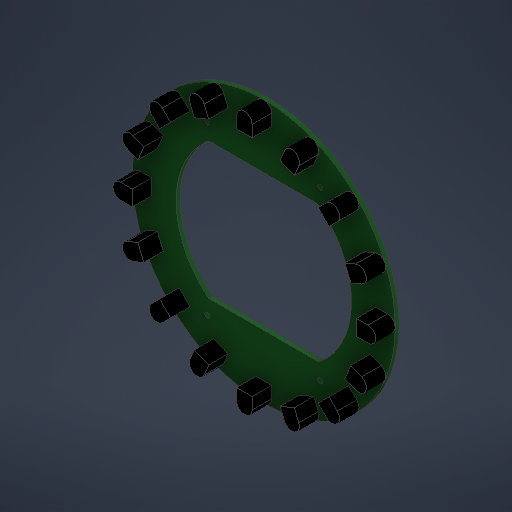
# Autodesk Inventor part: Main Board
Saved by Autodesk Inventor 2026.1 (Build 301233020, 233B)
## iProperties
Created: 2025-11-27
Part Number: Main Board
Material: Generic
Document SubType Name: Modeling
Designer: Bahaa
Density: 1 g/cm^3
Appearance: Default
Author: Bahaa
Autodesk Inventor part; units mm, degrees
ref_plane "YZ Plane" through (0, 0, 0) normal (1, 0, 0) x (0, 1, 0)
ref_plane "XZ Plane" through (0, 0, 0) normal (0, 1, 0) x (-1, 0, 0)
ref_plane "XY Plane" through (0, 0, 0) normal (0, 0, 1) x (1, 0, 0)
sketch "Sketch1" plane through (0, 0, 0) normal (0, 1, 0) x (-1, 0, 0)
  circle A0 centre (0, 0) radius 67.5
  line L0 (0, 0) -> (67.5, 0) construction
  line L1 (0, 0) -> (0, -67.5) construction
  circle A1 centre (0, 0) radius 45
  line L2 (0, 45) -> (0, 35)
  line L3 (0, 35) -> (-28.2843, 35)
  line L4 (0, 35) -> (28.2843, 35)
  line L5 (0, 0) -> (67.5, 0) construction
  line L6 (0, 0) -> (-45, 0) construction
  circle A2 centre (29, 43) radius 1.35
  circle A3 centre (-29, 43) radius 1.35
  circle A4 centre (29, -43) radius 1.35
  circle A5 centre (-29, -43) radius 1.35
  line L7 (0, -35) -> (-28.2843, -35)
  line L8 (0, -35) -> (28.2843, -35)
  point P0 (0, -45)
  dimension "d0" = 135
  dimension "d18" = 90
  dimension "d19" = 10
  dimension "d21" = 70
  dimension "d28" = 67.5
  dimension "d29" = 86
  dimension "d30" = 29
  dimension "d31" = 2.7
  constraints: 18 end point, 8 symmetric about line, 6 centre point, 6 point on circle, 4 coincident, 3 horizontal, 2 point on line, 2 vertical, 1 perpendicular, 3 other
  measures "d0" diameter of A0
  measures "d18" diameter of A1
  measures "d19" distance of L2.start L2.end
  measures "d21" diameter of L3 L0
  measures "d28" distance from line of L5.end L2
  measures "d29" diameter of point (29, 43) L0
  measures "d30" horizontal distance of point (0, 0) point (29, 43)
  measures "d31" diameter of A2
extrude "Extrusion1" add sketch "Sketch1" along normal blind 2 contours A0 | L4 L2 A1 | A1 L7 L8 | L2 L3 A1
sketch "Sketch2" plane through (0, 0, 0) normal (0, -1, 0) x (1, 0, 0)
  circle A0 centre (0, 0) radius 67.5 construction
  line L0 (67.5, 0) -> (62.5, 0) construction
  line L1 (57.5, 4) -> (63.5, 4)
  line L2 (67.5, 0) -> (67.5, 0)
  line L3 (63.5, -4) -> (57.5, -4)
  line L4 (57.5, -4) -> (57.5, 4)
  line L5 (57.5, 4) -> (67.5, -4) construction
  line L6 (67.5, 4) -> (57.5, -4) construction
  arc A1 (63.5, -4) -> (67.5, 0) centre (63.5, 0) ccw
  arc A2 (67.5, 0) -> (63.5, 4) centre (63.5, 0) ccw
  line L7 (62.3619, 25.8311) -> (57.7425, 23.9177) construction
  line L8 (51.5923, 25.6998) -> (57.1356, 27.9959)
  line L9 (62.3619, 25.8311) -> (62.3619, 25.8311)
  line L10 (60.1971, 20.6049) -> (54.6538, 18.3088)
  line L11 (54.6538, 18.3088) -> (51.5923, 25.6998)
  line L12 (51.5923, 25.6998) -> (63.8926, 22.1356) construction
  line L13 (60.8311, 29.5266) -> (54.6538, 18.3088) construction
  arc A3 (60.1971, 20.6049) -> (62.3619, 25.8311) centre (58.6664, 24.3004) ccw
  arc A4 (62.3619, 25.8311) -> (57.1356, 27.9959) centre (58.6664, 24.3004) ccw
  line L14 (47.7297, 47.7297) -> (44.1942, 44.1942) construction
  line L15 (37.8302, 43.4871) -> (42.0729, 47.7297)
  line L16 (47.7297, 47.7297) -> (47.7297, 47.7297)
  line L17 (47.7297, 42.0729) -> (43.4871, 37.8302)
  line L18 (43.4871, 37.8302) -> (37.8302, 43.4871)
  line L19 (37.8302, 43.4871) -> (50.5581, 44.9013) construction
  line L20 (44.9013, 50.5581) -> (43.4871, 37.8302) construction
  arc A5 (47.7297, 42.0729) -> (47.7297, 47.7297) centre (44.9013, 44.9013) ccw
  arc A6 (47.7297, 47.7297) -> (42.0729, 47.7297) centre (44.9013, 44.9013) ccw
  line L21 (25.8311, 62.3619) -> (23.9177, 57.7425) construction
  line L22 (18.3088, 54.6538) -> (20.6049, 60.1971)
  line L23 (25.8311, 62.3619) -> (25.8311, 62.3619)
  line L24 (27.9959, 57.1356) -> (25.6998, 51.5923)
  line L25 (25.6998, 51.5923) -> (18.3088, 54.6538)
  line L26 (18.3088, 54.6538) -> (29.5266, 60.8311) construction
  line L27 (22.1356, 63.8926) -> (25.6998, 51.5923) construction
  arc A7 (27.9959, 57.1356) -> (25.8311, 62.3619) centre (24.3004, 58.6664) ccw
  arc A8 (25.8311, 62.3619) -> (20.6049, 60.1971) centre (24.3004, 58.6664) ccw
  line L28 (0, 67.5) -> (0, 62.5) construction
  line L29 (-4, 57.5) -> (-4, 63.5)
  line L30 (0, 67.5) -> (0, 67.5)
  line L31 (4, 63.5) -> (4, 57.5)
  line L32 (4, 57.5) -> (-4, 57.5)
  line L33 (-4, 57.5) -> (4, 67.5) construction
  line L34 (-4, 67.5) -> (4, 57.5) construction
  arc A9 (4, 63.5) -> (0, 67.5) centre (0, 63.5) ccw
  arc A10 (0, 67.5) -> (-4, 63.5) centre (0, 63.5) ccw
  line L35 (-25.8311, 62.3619) -> (-23.9177, 57.7425) construction
  line L36 (-25.6998, 51.5923) -> (-27.9959, 57.1356)
  line L37 (-25.8311, 62.3619) -> (-25.8311, 62.3619)
  line L38 (-20.6049, 60.1971) -> (-18.3088, 54.6538)
  line L39 (-18.3088, 54.6538) -> (-25.6998, 51.5923)
  line L40 (-25.6998, 51.5923) -> (-22.1356, 63.8926) construction
  line L41 (-29.5266, 60.8311) -> (-18.3088, 54.6538) construction
  arc A11 (-20.6049, 60.1971) -> (-25.8311, 62.3619) centre (-24.3004, 58.6664) ccw
  arc A12 (-25.8311, 62.3619) -> (-27.9959, 57.1356) centre (-24.3004, 58.6664) ccw
  line L42 (-47.7297, 47.7297) -> (-44.1942, 44.1942) construction
  line L43 (-43.4871, 37.8302) -> (-47.7297, 42.0729)
  line L44 (-47.7297, 47.7297) -> (-47.7297, 47.7297)
  line L45 (-42.0729, 47.7297) -> (-37.8302, 43.4871)
  line L46 (-37.8302, 43.4871) -> (-43.4871, 37.8302)
  line L47 (-43.4871, 37.8302) -> (-44.9013, 50.5581) construction
  line L48 (-50.5581, 44.9013) -> (-37.8302, 43.4871) construction
  arc A13 (-42.0729, 47.7297) -> (-47.7297, 47.7297) centre (-44.9013, 44.9013) ccw
  arc A14 (-47.7297, 47.7297) -> (-47.7297, 42.0729) centre (-44.9013, 44.9013) ccw
  line L49 (-62.3619, 25.8311) -> (-57.7425, 23.9177) construction
  line L50 (-54.6538, 18.3088) -> (-60.1971, 20.6049)
  line L51 (-62.3619, 25.8311) -> (-62.3619, 25.8311)
  line L52 (-57.1356, 27.9959) -> (-51.5923, 25.6998)
  line L53 (-51.5923, 25.6998) -> (-54.6538, 18.3088)
  line L54 (-54.6538, 18.3088) -> (-60.8311, 29.5266) construction
  line L55 (-63.8926, 22.1356) -> (-51.5923, 25.6998) construction
  arc A15 (-57.1356, 27.9959) -> (-62.3619, 25.8311) centre (-58.6664, 24.3004) ccw
  arc A16 (-62.3619, 25.8311) -> (-60.1971, 20.6049) centre (-58.6664, 24.3004) ccw
  line L56 (-67.5, 0) -> (-62.5, 0) construction
  line L57 (-57.5, -4) -> (-63.5, -4)
  line L58 (-67.5, 0) -> (-67.5, 0)
  line L59 (-63.5, 4) -> (-57.5, 4)
  line L60 (-57.5, 4) -> (-57.5, -4)
  line L61 (-57.5, -4) -> (-67.5, 4) construction
  line L62 (-67.5, -4) -> (-57.5, 4) construction
  arc A17 (-63.5, 4) -> (-67.5, 0) centre (-63.5, 0) ccw
  arc A18 (-67.5, 0) -> (-63.5, -4) centre (-63.5, 0) ccw
  line L63 (-62.3619, -25.8311) -> (-57.7425, -23.9177) construction
  line L64 (-51.5923, -25.6998) -> (-57.1356, -27.9959)
  line L65 (-62.3619, -25.8311) -> (-62.3619, -25.8311)
  line L66 (-60.1971, -20.6049) -> (-54.6538, -18.3088)
  line L67 (-54.6538, -18.3088) -> (-51.5923, -25.6998)
  line L68 (-51.5923, -25.6998) -> (-63.8926, -22.1356) construction
  line L69 (-60.8311, -29.5266) -> (-54.6538, -18.3088) construction
  arc A19 (-60.1971, -20.6049) -> (-62.3619, -25.8311) centre (-58.6664, -24.3004) ccw
  arc A20 (-62.3619, -25.8311) -> (-57.1356, -27.9959) centre (-58.6664, -24.3004) ccw
  line L70 (-47.7297, -47.7297) -> (-44.1942, -44.1942) construction
  line L71 (-37.8302, -43.4871) -> (-42.0729, -47.7297)
  line L72 (-47.7297, -47.7297) -> (-47.7297, -47.7297)
  line L73 (-47.7297, -42.0729) -> (-43.4871, -37.8302)
  line L74 (-43.4871, -37.8302) -> (-37.8302, -43.4871)
  line L75 (-37.8302, -43.4871) -> (-50.5581, -44.9013) construction
  line L76 (-44.9013, -50.5581) -> (-43.4871, -37.8302) construction
  arc A21 (-47.7297, -42.0729) -> (-47.7297, -47.7297) centre (-44.9013, -44.9013) ccw
  arc A22 (-47.7297, -47.7297) -> (-42.0729, -47.7297) centre (-44.9013, -44.9013) ccw
  line L77 (-25.8311, -62.3619) -> (-23.9177, -57.7425) construction
  line L78 (-18.3088, -54.6538) -> (-20.6049, -60.1971)
  line L79 (-25.8311, -62.3619) -> (-25.8311, -62.3619)
  line L80 (-27.9959, -57.1356) -> (-25.6998, -51.5923)
  line L81 (-25.6998, -51.5923) -> (-18.3088, -54.6538)
  line L82 (-18.3088, -54.6538) -> (-29.5266, -60.8311) construction
  line L83 (-22.1356, -63.8926) -> (-25.6998, -51.5923) construction
  arc A23 (-27.9959, -57.1356) -> (-25.8311, -62.3619) centre (-24.3004, -58.6664) ccw
  arc A24 (-25.8311, -62.3619) -> (-20.6049, -60.1971) centre (-24.3004, -58.6664) ccw
  line L84 (0, -67.5) -> (0, -62.5) construction
  line L85 (4, -57.5) -> (4, -63.5)
  line L86 (0, -67.5) -> (0, -67.5)
  line L87 (-4, -63.5) -> (-4, -57.5)
  line L88 (-4, -57.5) -> (4, -57.5)
  line L89 (4, -57.5) -> (-4, -67.5) construction
  line L90 (4, -67.5) -> (-4, -57.5) construction
  arc A25 (-4, -63.5) -> (0, -67.5) centre (0, -63.5) ccw
  arc A26 (0, -67.5) -> (4, -63.5) centre (0, -63.5) ccw
  line L91 (25.8311, -62.3619) -> (23.9177, -57.7425) construction
  line L92 (25.6998, -51.5923) -> (27.9959, -57.1356)
  line L93 (25.8311, -62.3619) -> (25.8311, -62.3619)
  line L94 (20.6049, -60.1971) -> (18.3088, -54.6538)
  line L95 (18.3088, -54.6538) -> (25.6998, -51.5923)
  line L96 (25.6998, -51.5923) -> (22.1356, -63.8926) construction
  line L97 (29.5266, -60.8311) -> (18.3088, -54.6538) construction
  arc A27 (20.6049, -60.1971) -> (25.8311, -62.3619) centre (24.3004, -58.6664) ccw
  arc A28 (25.8311, -62.3619) -> (27.9959, -57.1356) centre (24.3004, -58.6664) ccw
  line L98 (47.7297, -47.7297) -> (44.1942, -44.1942) construction
  line L99 (43.4871, -37.8302) -> (47.7297, -42.0729)
  line L100 (47.7297, -47.7297) -> (47.7297, -47.7297)
  line L101 (42.0729, -47.7297) -> (37.8302, -43.4871)
  line L102 (37.8302, -43.4871) -> (43.4871, -37.8302)
  line L103 (43.4871, -37.8302) -> (44.9013, -50.5581) construction
  line L104 (50.5581, -44.9013) -> (37.8302, -43.4871) construction
  arc A29 (42.0729, -47.7297) -> (47.7297, -47.7297) centre (44.9013, -44.9013) ccw
  arc A30 (47.7297, -47.7297) -> (47.7297, -42.0729) centre (44.9013, -44.9013) ccw
  line L105 (62.3619, -25.8311) -> (57.7425, -23.9177) construction
  line L106 (54.6538, -18.3088) -> (60.1971, -20.6049)
  line L107 (62.3619, -25.8311) -> (62.3619, -25.8311)
  line L108 (57.1356, -27.9959) -> (51.5923, -25.6998)
  line L109 (51.5923, -25.6998) -> (54.6538, -18.3088)
  line L110 (54.6538, -18.3088) -> (60.8311, -29.5266) construction
  line L111 (63.8926, -22.1356) -> (51.5923, -25.6998) construction
  arc A31 (57.1356, -27.9959) -> (62.3619, -25.8311) centre (58.6664, -24.3004) ccw
  arc A32 (62.3619, -25.8311) -> (60.1971, -20.6049) centre (58.6664, -24.3004) ccw
  point P0 (-47.7297, -47.7297)
  point P1 (62.3619, 25.8311)
  point P2 (-62.3619, -25.8311)
  point P3 (-62.3619, 25.8311)
  point P4 (0, 67.5)
  point P5 (-47.7297, 47.7297)
  point P6 (-25.8311, 62.3619)
  point P7 (-25.8311, -62.3619)
  point P8 (25.8311, 62.3619)
  point P9 (-67.5, 0)
  point P10 (62.3619, -25.8311)
  point P11 (25.8311, -62.3619)
  point P12 (0, -67.5)
  dimension "d7" = 5
  dimension "d8" = 10
  dimension "d9" = 8
  dimension "d10" = 4
  dimension "d13" = 360
  constraints: 224 end point, 64 point on circle, 64 point on line, 32 centre point, 4 tangent, 2 horizontal, 2 midpoint, 2 parallel, 1 concentric, 1 horizontal alignment, 1 perpendicular, 1 vertical, 338 other
  measures "d7" distance of L0.start L0.end
  measures "d8" distance of L5.end L3.end
  measures "d9" distance of L3.end L1.start
  measures "d10" radius of A1
extrude "Extrusion2" add sketch "Sketch2" along normal blind 10
fillet "Fillet1" radius 5 2 edges at (-28.2843, 1, 35) (28.2843, 1, 35)
equation "\"d28\" = 0.5 * d0"
body "Solid1"
